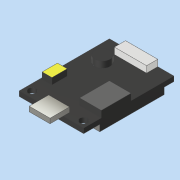
# Autodesk Inventor part: VideoTransmitter
Saved by Autodesk Inventor 2017.3 (Build 213256000, 256)
## iProperties
Created: 2018-07-15
Part Number: VideoTransmitter
Material: ABS Plastic
Document SubType Name: Modeling
Designer: Derek Wider
Density: 1.06 g/cm^3
Appearance: Smooth - Black
Author: Derek Wider
Autodesk Inventor part; units mm, degrees
ref_plane "YZ Plane" through (0, 0, 0) normal (1, 0, 0) x (0, 1, 0)
ref_plane "XZ Plane" through (0, 0, 0) normal (0, 1, 0) x (-1, 0, 0)
ref_plane "XY Plane" through (0, 0, 0) normal (0, 0, 1) x (1, 0, 0)
sketch "Sketch1" plane through (0, 0, 0) normal (0, 1, 0) x (-1, 0, 0)
  line L0 (0, 0) -> (20, 0)
  line L1 (20, 0) -> (20, -28)
  line L2 (20, -28) -> (0, -28)
  line L3 (0, -28) -> (0, 0)
  dimension "d0" = 28
  dimension "d1" = 20
  constraints: 8 end point, 2 parallel, 1 horizontal, 1 perpendicular
  measures "d0" distance of L2.end L0.start
  measures "d1" distance of L0.start L0.end
extrude "Extrusion1" add sketch "Sketch1" along normal blind 1.5
sketch "Sketch2" plane through (0, 1.5, 0) normal (0, 1, 0) x (1, 0, 0)
  line L0 (0, 28) -> (-20, 28) projected
  line L1 (-5, 28) -> (-15, 28)
  line L2 (-15, 28) -> (-15, 24.5354)
  line L3 (-15, 24.5354) -> (-5, 24.5354)
  line L4 (-5, 24.5354) -> (-5, 28)
  point P0 (0, 0)
  point P1 (-10, 24.5354)
  point P2 (-10, 28)
  dimension "d4" = 10
  constraints: 8 end point, 2 midpoint, 2 parallel, 1 horizontal, 1 perpendicular, 1 point on line, 1 vertical alignment
  measures "d4" distance of L2.end L3.end
extrude "Extrusion2" add sketch "Sketch2" along normal blind 2
sketch "Sketch3" plane through (0, 1.5, 0) normal (0, 1, 0) x (1, 0, 0)
  line L0 (0, 0) -> (0, 28) projected
  line L1 (0, 5.4716) -> (-6.7562, 5.4716)
  line L2 (-6.7562, 5.4716) -> (-6.7562, 14.73)
  line L3 (-6.7562, 14.73) -> (0, 14.73)
  line L4 (0, 14.73) -> (0, 5.4716)
  constraints: 8 end point, 2 parallel, 1 horizontal, 1 perpendicular, 1 point on line
extrude "Extrusion3" add sketch "Sketch3" along normal blind 2
sketch "Sketch4" plane through (0, 1.5, 0) normal (0, 1, 0) x (1, 0, 0)
  circle A0 centre (-14.8135, 20.6337) radius 2.3748
  point P0 (0, 0)
  constraints: 1 centre point
extrude "Extrusion4" add sketch "Sketch4" along normal blind 2
sketch "Sketch5" plane through (0, 1.5, 0) normal (0, 1, 0) x (1, 0, 0)
  circle A0 centre (-2, 2) radius 1.25
  circle A1 centre (-18, 2) radius 1.25
  line L0 (0, 0) -> (0, 5.4716) projected
  line L1 (-20, 0) -> (0, 0) projected
  line L2 (-20, 28) -> (-20, 0) projected
  dimension "d11" = 2
  dimension "d12" = 2.5
  dimension "d13" = 2
  dimension "d14" = 2
  dimension "d15" = 2
  dimension "d16" = 2.5
  constraints: 2 centre point
  measures "d11" distance from line of L0 A0.centre
  measures "d12" diameter of A0
  measures "d13" distance from line of A0.centre L1
  measures "d14" distance from line of L2 A1.centre
  measures "d15" distance from line of A1.centre L1
  measures "d16" diameter of A1
extrude "Extrusion5" cut sketch "Sketch5" against normal blind 2
sketch "Sketch6" plane through (0, 0, 0) normal (0, -1, 0) x (1, 0, 0)
  line L0 (-20, 0) -> (-20, -28) projected
  line L1 (-20, -25) -> (0, -25)
  line L2 (0, -25) -> (0, -5)
  line L3 (0, -5) -> (-20, -5)
  line L4 (-20, -5) -> (-20, -25)
  line L5 (-20, -28) -> (0, -28) projected
  line L6 (0, 0) -> (-20, 0) projected
  dimension "d19" = 3
  dimension "d20" = 5
  constraints: 8 end point, 2 parallel, 1 horizontal, 1 perpendicular, 1 point on line
  measures "d19" distance between parallel lines of L5 L1
  measures "d20" distance between parallel lines of L6 L3
extrude "Extrusion6" add sketch "Sketch6" along normal blind 2
sketch "Sketch7" plane through (0, 1.5, 0) normal (0, 1, 0) x (1, 0, 0)
  line L0 (-16.4979, 6.6511) -> (-19.5294, 6.6511)
  line L1 (-19.5294, 6.6511) -> (-19.5294, 11.4005)
  line L2 (-19.5294, 11.4005) -> (-16.4979, 11.4005)
  line L3 (-16.4979, 11.4005) -> (-16.4979, 6.6511)
  point P0 (0, 0)
  constraints: 8 end point, 2 parallel, 1 horizontal, 1 perpendicular
extrude "Extrusion7" add sketch "Sketch7" along normal blind 2
sketch "Sketch8" plane through (0, 1.5, 0) normal (0, 1, 0) x (1, 0, 0)
  line L0 (-12.8387, 1.9896) -> (-6.3724, 1.9896)
  line L1 (-6.3724, 1.9896) -> (-6.3724, -4.0656)
  line L2 (-6.3724, -4.0656) -> (-12.8387, -4.0656)
  line L3 (-12.8387, -4.0656) -> (-12.8387, 1.9896)
  point P0 (0, 0)
  constraints: 8 end point, 2 parallel, 1 horizontal, 1 perpendicular
extrude "Extrusion8" add sketch "Sketch8" along normal blind 1.5
equation "\"d16\" = d12"
body "Solid1"
